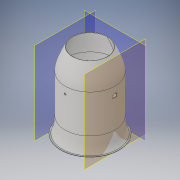
# Autodesk Inventor part: BrImp_Casing_v01
Saved by Autodesk Inventor 2018 (Build 220112000, 112)
## iProperties
Created: 2018-02-04
Part Number: BrImp_Casing_v01
Material: Generic
Document SubType Name: Modeling
Designer: Benedikt
Density: 1 g/cm^3
Appearance: Default
Author: Benedikt
## iProperties of the stored document BrImp_Casing_v01_3DPrint.ipt
Created: 2018-02-04
Part Number: BrImp_Casing_v01_3DPrint
Material: Generic
Document SubType Name: Modeling
Designer: Benedikt
Density: 1 g/cm^3
Appearance: Default
Author: Benedikt
Autodesk Inventor part; units mm, degrees
ref_plane "YZ Plane" through (0, 0, 0) normal (1, 0, 0) x (0, 1, 0)
ref_plane "XZ Plane" through (0, 0, 0) normal (0, 1, 0) x (-1, 0, 0)
ref_plane "XY Plane" through (0, 0, 0) normal (0, 0, 1) x (1, 0, 0)
sketch "Sketch1" plane through (0, 0, 0) normal (1, 0, 0) x (0, 1, 0)
  line L0 (45, 10) -> (45, -60)
  line L1 (45, -60) -> (45, -81.6721) construction
  line L2 (45, -81.6721) -> (50.517, -88.3707) construction
  spline S0 degree 2 poles (45, -60) (45, -81.6721) (50.517, -88.3707) knots 1 1 1 2 2 2
  line L3 (0, 67.9848) -> (0, -121.7478) construction
  line L4 (45, 10) -> (45, 18.486) construction
  line L5 (45, 18.486) -> (41.9833, 28.8243) construction
  line L6 (41.9833, 28.8243) -> (31.6199, 50) construction
  spline S1 degree 3 poles (45, 10) (45, 18.486) (41.9833, 28.8243) (31.6199, 50) knots 1 1 1 1 2 2 2 2
  line L7 (45.8, -60) -> (45.8, 10)
  line L8 (32.3384, 50.3517) -> (31.6199, 50)
  line L9 (50.517, -88.3707) -> (53.517, -88.3707)
  line L10 (53.517, -88.3707) -> (53.517, -87.8621)
  line L11 (53.517, -87.8621) -> (51.1345, -87.8621)
  spline S2 degree 5 poles (51.1345, -87.8621) (50.2967, -86.845) (49.6263, -85.693) (49.075, -84.4931) (47.9413, -81.4774) (47.2186, -78.3345) (46.8812, -76.4648) (46.2611, -72.0638) (45.9532, -67.6291) (45.8477, -65.087) (45.8, -62.5435) (45.8, -60) knots 0 0 0 0 0 0 0.228736 0.228736 0.228736 0.55838 0.55838 0.55838 1 1 1 1 1 1
  spline S3 degree 5 poles (45.8, 10) (45.8001, 11.9423) (45.6709, 13.8852) (45.4119, 15.8148) (44.5559, 20.3736) (43.2383, 24.825) (42.3723, 27.375) (40.0583, 33.592) (37.4063, 39.6738) (35.7643, 43.2555) (34.0702, 46.8129) (32.3384, 50.3517) knots 0 0 0 0 0 0 0.226541 0.226541 0.226541 0.540496 0.540496 0.540496 1 1 1 1 1 1
  point P0 (0, 0)
  dimension "d0" = 45
  dimension "d1" = 70
  dimension "d4" = 10
  dimension "d7" = 40
  dimension "d9" = 0.8
  dimension "d28" = 3
  constraints: 14 end point, 4 vertical, 3 perpendicular, 2 parallel, 1 horizontal, 12 other
  measures "d0" distance from line of L0 point (0, 0)
  measures "d1" distance of L0.start L0.end
  measures "d4" vertical distance of point (0, 0) L0.start
  measures "d7" vertical distance of L6.end L0.start
  measures "d9" distance between parallel lines of L0 L7
  measures "d28" distance of L2.end L9.end
revolve "Revolution3" add sketch "Sketch1" angle 360 about axis through (0, 0, 67.9848) along (0, 0, -1)
ref_plane "Work Plane2" through (0, 45.8, -25) normal (0, 1, 0) x (-1, 0, 0)
ref_plane "Work Plane1" through (3.7, 14.1, -14) normal (0, 1, 0) x (-1, 0, 0)
ref_plane "Work Plane4" through (-45.8, 0, -25) normal (-1, 0, 0) x (0, -1, 0)
ref_plane "Work Plane3" through (-14.1, 3.7, -14) normal (-1, 0, 0) x (0, 0, 1)
sketch "Sketch2" plane through (-45.8, 0, -25) normal (-1, 0, 0) x (0, -1, 0)
  circle A0 centre (0, 22.5) radius 1.7
  point P0 (0, 25)
  constraints: 1 centre point, 1 coincident
hole "Hole1" at (-45.8, 0, -2.5) direction (1, 0, 0) diameter 3.4 end through all
sketch "Sketch3" plane through (0, 45.8, -25) normal (0, 1, 0) x (-1, 0, 0)
  circle A0 centre (0, 22.5) radius 1.7
  point P0 (0, 25)
  constraints: 1 centre point
hole "Hole2" at (0, 45.8, -2.5) direction (0, -1, 0) diameter 3.4 end through all
ref_plane "Work Plane6" through (45.8, 0, -25) normal (1, 0, 0) x (0, 1, 0)
ref_plane "Work Plane5" through (14.1, -3.7, -14) normal (1, 0, 0) x (0, 0, -1)
sketch "Sketch4" plane through (45.8, 0, -25) normal (1, 0, 0) x (0, 1, 0)
  line L0 (-4, 22) -> (4, 22) projected
  line L1 (-4, 22) -> (-4, 17)
  line L2 (-4, 17) -> (4, 17)
  line L3 (4, 17) -> (4, 22)
  point P0 (0, 25)
  dimension "d25" = 5
  constraints: 6 end point, 2 perpendicular, 1 vertical
  measures "d25" distance of L0.start L1.end
extrude "Extrusion1" cut sketch "Sketch4" against normal blind 2.75
body "Solid3"
